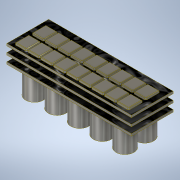
# Autodesk Inventor part: UberDriver_0
Saved by Autodesk Inventor 2020 (Build 240168000, 168)
## iProperties
Created: 2019-02-21
Part Number: UberDriver_0
Material: Silver
Document SubType Name: Modeling
Designer: atmat
Density: 10.49 g/cm^3
Appearance: Silver
Mass: 97.9587 g
Surface Area: 98.3282 cm^2
Volume: 9.3383 cm^3
Author: atmat
Autodesk Inventor part; units mm, degrees
ref_plane "YZ Plane" through (0, 0, 0) normal (1, 0, 0) x (0, 1, 0)
ref_plane "XZ Plane" through (0, 0, 0) normal (0, 1, 0) x (-1, 0, 0)
ref_plane "XY Plane" through (0, 0, 0) normal (0, 0, 1) x (1, 0, 0)
sketch "Szkic1" plane through (0, 0, 0) normal (0, 1, 0) x (-1, 0, 0)
  line L0 (27.94, 9.365) -> (-27.94, 9.365)
  line L1 (-27.94, 9.365) -> (-27.94, -9.365)
  line L2 (-27.94, -9.365) -> (27.94, -9.365)
  line L3 (27.94, -9.365) -> (27.94, 9.365)
  point P0 (0, 0)
  dimension "d0" = 18.73
  dimension "d1" = 9.365
  dimension "d2" = 55.88
  dimension "d3" = 27.94
  constraints: 8 end point, 2 parallel, 1 horizontal, 1 perpendicular
  measures "d0" distance of L2.end L0.start
  measures "d1" distance from line of L0 point (0, 0)
  measures "d2" distance of L0.start L0.end
  measures "d3" distance from line of point (0, 0) L3
extrude "Wyciągnięcie proste1" add sketch "Szkic1" along normal blind 1
sketch "Szkic2" plane through (0, 1, 0) normal (0, 1, 0) x (1, 0, 0)
  line L0 (-25.4, -8.095) -> (-20.32, -8.095)
  line L1 (-20.32, -8.095) -> (-20.32, -2.065)
  line L2 (-20.32, -2.065) -> (-25.4, -2.065)
  line L3 (-25.4, -2.065) -> (-25.4, -8.095)
  line L4 (-27.94, 9.365) -> (-27.94, -9.365) projected
  line L5 (-27.94, -9.365) -> (27.94, -9.365) projected
  line L6 (-19.68, -8.095) -> (-14.6, -8.095)
  line L7 (-14.6, -8.095) -> (-14.6, -2.065)
  line L8 (-14.6, -2.065) -> (-19.68, -2.065)
  line L9 (-19.68, -2.065) -> (-19.68, -8.095)
  line L10 (-13.96, -8.095) -> (-8.88, -8.095)
  line L11 (-8.88, -8.095) -> (-8.88, -2.065)
  line L12 (-8.88, -2.065) -> (-13.96, -2.065)
  line L13 (-13.96, -2.065) -> (-13.96, -8.095)
  line L14 (-8.24, -8.095) -> (-3.16, -8.095)
  line L15 (-3.16, -8.095) -> (-3.16, -2.065)
  line L16 (-3.16, -2.065) -> (-8.24, -2.065)
  line L17 (-8.24, -2.065) -> (-8.24, -8.095)
  line L18 (-2.52, -8.095) -> (2.56, -8.095)
  line L19 (2.56, -8.095) -> (2.56, -2.065)
  line L20 (2.56, -2.065) -> (-2.52, -2.065)
  line L21 (-2.52, -2.065) -> (-2.52, -8.095)
  line L22 (3.2, -8.095) -> (8.28, -8.095)
  line L23 (8.28, -8.095) -> (8.28, -2.065)
  line L24 (8.28, -2.065) -> (3.2, -2.065)
  line L25 (3.2, -2.065) -> (3.2, -8.095)
  line L26 (8.92, -8.095) -> (14, -8.095)
  line L27 (14, -8.095) -> (14, -2.065)
  line L28 (14, -2.065) -> (8.92, -2.065)
  line L29 (8.92, -2.065) -> (8.92, -8.095)
  line L30 (14.64, -8.095) -> (19.72, -8.095)
  line L31 (19.72, -8.095) -> (19.72, -2.065)
  line L32 (19.72, -2.065) -> (14.64, -2.065)
  line L33 (14.64, -2.065) -> (14.64, -8.095)
  line L34 (20.36, -8.095) -> (25.44, -8.095)
  line L35 (25.44, -8.095) -> (25.44, -2.065)
  line L36 (25.44, -2.065) -> (20.36, -2.065)
  line L37 (20.36, -2.065) -> (20.36, -8.095)
  line L38 (-25.4, -0.475) -> (-20.32, -0.475)
  line L39 (-20.32, -0.475) -> (-20.32, 5.555)
  line L40 (-20.32, 5.555) -> (-25.4, 5.555)
  line L41 (-25.4, 5.555) -> (-25.4, -0.475)
  line L42 (-19.68, -0.475) -> (-14.6, -0.475)
  line L43 (-14.6, -0.475) -> (-14.6, 5.555)
  line L44 (-14.6, 5.555) -> (-19.68, 5.555)
  line L45 (-19.68, 5.555) -> (-19.68, -0.475)
  line L46 (-13.96, -0.475) -> (-8.88, -0.475)
  line L47 (-8.88, -0.475) -> (-8.88, 5.555)
  line L48 (-8.88, 5.555) -> (-13.96, 5.555)
  line L49 (-13.96, 5.555) -> (-13.96, -0.475)
  line L50 (19.72, 5.555) -> (14.64, 5.555)
  line L51 (19.72, -0.475) -> (19.72, 5.555)
  line L52 (14.64, -0.475) -> (19.72, -0.475)
  line L53 (14.64, 5.555) -> (14.64, -0.475)
  line L54 (25.44, 5.555) -> (20.36, 5.555)
  line L55 (25.44, -0.475) -> (25.44, 5.555)
  line L56 (20.36, -0.475) -> (25.44, -0.475)
  line L57 (20.36, 5.555) -> (20.36, -0.475)
  line L58 (-3.16, 5.555) -> (-8.24, 5.555)
  line L59 (-3.16, -0.475) -> (-3.16, 5.555)
  line L60 (-8.24, -0.475) -> (-3.16, -0.475)
  line L61 (-8.24, 5.555) -> (-8.24, -0.475)
  line L62 (2.56, 5.555) -> (-2.52, 5.555)
  line L63 (2.56, -0.475) -> (2.56, 5.555)
  line L64 (-2.52, -0.475) -> (2.56, -0.475)
  line L65 (-2.52, 5.555) -> (-2.52, -0.475)
  line L66 (8.28, 5.555) -> (3.2, 5.555)
  line L67 (8.28, -0.475) -> (8.28, 5.555)
  line L68 (3.2, -0.475) -> (8.28, -0.475)
  line L69 (3.2, 5.555) -> (3.2, -0.475)
  line L70 (14, 5.555) -> (8.92, 5.555)
  line L71 (14, -0.475) -> (14, 5.555)
  line L72 (8.92, -0.475) -> (14, -0.475)
  line L73 (8.92, 5.555) -> (8.92, -0.475)
  point P0 (0, 0)
  dimension "d6" = 6.03
  dimension "d7" = 5.08
  dimension "d8" = 2.54
  dimension "d9" = 1.27
  dimension "d10" = 5.08
  dimension "d11" = 6.03
  dimension "d12" = 1.27
  dimension "d13" = 0.64
  dimension "d14" = 5.08
  dimension "d15" = 6.03
  dimension "d16" = 1.27
  dimension "d17" = 0.64
  dimension "d18" = 5.08
  dimension "d19" = 6.03
  dimension "d20" = 1.27
  dimension "d21" = 0.64
  dimension "d22" = 5.08
  dimension "d23" = 6.03
  dimension "d24" = 1.27
  dimension "d25" = 0.64
  dimension "d26" = 5.08
  dimension "d27" = 6.03
  dimension "d28" = 5.08
  dimension "d29" = 6.03
  dimension "d30" = 5.08
  dimension "d31" = 6.03
  dimension "d32" = 5.08
  dimension "d33" = 6.03
  dimension "d34" = 0.64
  dimension "d35" = 0.64
  dimension "d36" = 0.64
  dimension "d37" = 0.64
  dimension "d38" = 1.27
  dimension "d39" = 1.27
  dimension "d40" = 1.27
  dimension "d41" = 1.27
  dimension "d42" = 6.03
  dimension "d43" = 5.08
  dimension "d44" = 6.03
  dimension "d45" = 5.08
  dimension "d46" = 6.03
  dimension "d47" = 5.08
  dimension "d48" = 1.59
  dimension "d49" = 0
  dimension "d50" = 0
  dimension "d51" = 0
  dimension "d52" = 0
  dimension "d53" = 0
  dimension "d54" = 5.08
  dimension "d55" = 6.03
  dimension "d56" = 5.08
  dimension "d57" = 6.03
  dimension "d58" = 0.64
  dimension "d59" = 0
  dimension "d60" = 0
  dimension "d61" = 0
  dimension "d62" = 5.08
  dimension "d63" = 6.03
  dimension "d64" = 5.08
  dimension "d65" = 6.03
  dimension "d66" = 0.64
  dimension "d67" = 0
  dimension "d68" = 0
  dimension "d69" = 0
  constraints: 144 end point, 36 parallel, 18 horizontal, 18 perpendicular
  measures "d6" distance of L2.end L0.start
  measures "d7" distance of L1.end L2.end
  measures "d8" distance between parallel lines of L4 L3
  measures "d9" distance between parallel lines of L5 L0
  measures "d10" distance of L7.end L8.end
  measures "d11" distance of L8.end L6.start
  measures "d12" distance between parallel lines of L5 L6
  measures "d13" distance between parallel lines of L9 L1
  measures "d14" distance of L12.start L12.end
  measures "d15" distance of L12.end L10.start
  measures "d16" distance between parallel lines of L5 L10
  measures "d17" distance between parallel lines of L13 L7
  measures "d18" distance of L16.start L16.end
  measures "d19" distance of L16.end L14.start
  measures "d20" distance between parallel lines of L14 L5
  measures "d21" distance between parallel lines of L11 L17
  measures "d22" distance of L20.start L20.end
  measures "d23" distance of L20.end L18.start
  measures "d24" distance between parallel lines of L5 L18
  measures "d25" distance between parallel lines of L15 L21
  measures "d26" distance of L24.start L24.end
  measures "d27" distance of L24.end L22.start
  measures "d28" distance of L28.start L28.end
  measures "d29" distance of L28.end L26.start
  measures "d30" distance of L32.start L32.end
  measures "d31" distance of L32.end L30.start
  measures "d32" distance of L36.start L36.end
  measures "d33" distance of L36.end L34.start
  measures "d34" distance between parallel lines of L25 L19
  measures "d35" distance between parallel lines of L29 L23
  measures "d36" distance between parallel lines of L33 L27
  measures "d37" distance between parallel lines of L37 L31
  measures "d38" distance between parallel lines of L5 L22
  measures "d39" distance between parallel lines of L5 L26
  measures "d40" distance between parallel lines of L5 L30
  measures "d41" distance between parallel lines of L5 L34
  measures "d42" distance of L40.end L38.start
  measures "d43" distance of L39.end L40.end
  measures "d44" distance of L44.end L42.start
  measures "d45" distance of L43.end L44.end
  measures "d46" distance of L48.end L46.start
  measures "d47" distance of L47.end L48.end
  measures "d48" distance between parallel lines of L38 L2
  measures "d49" distance between parallel lines of L3 L41
  measures "d50" distance between parallel lines of L9 L45
  measures "d51" distance between parallel lines of L13 L49
  measures "d52" distance between parallel lines of L38 L42
  measures "d53" distance between parallel lines of L42 L46
  measures "d54" distance of L50.start L53.start
  measures "d55" distance of L53.start L53.end
  measures "d56" distance of L54.start L57.start
  measures "d57" distance of L57.start L57.end
  measures "d58" distance between parallel lines of L57 L51
  measures "d59" distance between parallel lines of L52 L46
  measures "d60" distance between parallel lines of L52 L56
  measures "d61" distance between parallel lines of L37 L57
  measures "d62" distance of L58.start L61.start
  measures "d63" distance of L61.start L61.end
  measures "d64" distance of L62.start L65.start
  measures "d65" distance of L65.start L65.end
  measures "d66" distance between parallel lines of L65 L59
  measures "d67" distance between parallel lines of L58 L62
  measures "d68" distance between parallel lines of L19 L63
  measures "d69" distance between parallel lines of L48 L58
extrude "Wyciągnięcie proste2" add sketch "Szkic2" along normal blind 1
chamfer "Faza1" distance 0.2 angle 45 4 edges at (22.9, 2, 8.095) (25.44, 2, 5.08) (20.36, 2, 5.08) (22.9, 2, 2.065)
chamfer "Faza2" distance 0.2 angle 45 68 edges at (17.18, 2, 8.095) (19.72, 2, 5.08) (14.64, 2, 5.08) (17.18, 2, 2.065) (14, 2, 5.08) (11.46, 2, 8.095) (8.92, 2, 5.08) (11.46, 2, 2.065) (8.28, 2, 5.08) (5.74, 2, 8.095) (3.2, 2, 5.08) (5.74, 2, 2.065) (0.02, 2, 8.095) (-5.7, 2, 8.095) (-11.42, 2, 8.095) (-17.14, 2, 8.095) (-22.86, 2, 8.095) (-25.4, 2, 5.08) (-22.86, 2, 2.065) (-17.14, 2, 2.065) (-19.68, 2, 5.08) (-14.6, 2, 5.08) (-13.96, 2, 5.08) (-8.88, 2, 5.08) (-11.42, 2, 2.065) (-5.7, 2, 2.065) (-3.16, 2, 5.08) (-8.24, 2, 5.08) (-20.32, 2, 5.08) (-20.32, 2, -2.54) (-22.86, 2, 0.475) (-25.4, 2, -2.54) (-22.86, 2, -5.555) (-17.14, 2, -5.555) (-19.68, 2, -2.54) (-17.14, 2, 0.475) (-14.6, 2, -2.54) (-11.42, 2, 0.475) (-13.96, 2, -2.54) (-11.42, 2, -5.555) (-8.88, 2, -2.54) (-5.7, 2, 0.475) (-8.24, 2, -2.54) (-5.7, 2, -5.555) (-3.16, 2, -2.54) (0.02, 2, 2.065) (-2.52, 2, 5.08) (0.02, 2, 0.475) (-2.52, 2, -2.54) (0.02, 2, -5.555) (2.56, 2, -2.54) (5.74, 2, 0.475) (3.2, 2, -2.54) (5.74, 2, -5.555) (8.28, 2, -2.54) (11.46, 2, 0.475) (8.92, 2, -2.54) (11.46, 2, -5.555) (14, 2, -2.54) (17.18, 2, 0.475) (17.18, 2, -5.555) (14.64, 2, -2.54) (19.72, 2, -2.54) (22.9, 2, 0.475) (20.36, 2, -2.54) (22.9, 2, -5.555) (25.44, 2, -2.54) (2.56, 2, 5.08)
chamfer "Faza3" distance 0.5 angle 45 18 edges at (25.44, 1.4, 8.095) (19.72, 1.4, 8.095) (14, 1.4, 8.095) (8.28, 1.4, 8.095) (2.56, 1.4, 8.095) (2.56, 1.4, 0.475) (8.28, 1.4, 0.475) (14, 1.4, 0.475) (19.72, 1.4, 0.475) (25.44, 1.4, 0.475) (-3.16, 1.4, 0.475) (-3.16, 1.4, 8.095) (-8.88, 1.4, 8.095) (-14.6, 1.4, 8.095) (-8.88, 1.4, 0.475) (-14.6, 1.4, 0.475) (-20.32, 1.4, 0.475) (-20.32, 1.4, 8.095)
sketch "Szkic3" plane through (0, 0, 0) normal (0, -1, 0) x (1, 0, 0)
  line L0 (-25.08, -2.085) -> (-21.9, -2.085)
  line L1 (-21.9, -2.085) -> (-21.9, -8.435)
  line L2 (-21.9, -8.435) -> (-25.08, -8.435)
  line L3 (-25.08, -8.435) -> (-25.08, -2.085)
  line L4 (-25.4, 0.475) -> (-25.4, -5.555) projected
  line L5 (27.94, -9.365) -> (-27.94, -9.365) projected
  line L6 (-19.36, -2.085) -> (-16.18, -2.085)
  line L7 (-16.18, -2.085) -> (-16.18, -8.435)
  line L8 (-16.18, -8.435) -> (-19.36, -8.435)
  line L9 (-19.36, -8.435) -> (-19.36, -2.085)
  line L10 (-19.68, 0.475) -> (-19.68, -5.555) projected
  line L11 (-13.64, -2.085) -> (-10.46, -2.085)
  line L12 (-10.46, -2.085) -> (-10.46, -8.435)
  line L13 (-10.46, -8.435) -> (-13.64, -8.435)
  line L14 (-13.64, -8.435) -> (-13.64, -2.085)
  line L15 (-7.92, -2.085) -> (-4.74, -2.085)
  line L16 (-4.74, -2.085) -> (-4.74, -8.435)
  line L17 (-4.74, -8.435) -> (-7.92, -8.435)
  line L18 (-7.92, -8.435) -> (-7.92, -2.085)
  line L19 (-2.2, -2.085) -> (0.98, -2.085)
  line L20 (0.98, -2.085) -> (0.98, -8.435)
  line L21 (0.98, -8.435) -> (-2.2, -8.435)
  line L22 (-2.2, -8.435) -> (-2.2, -2.085)
  line L23 (3.52, -2.085) -> (6.7, -2.085)
  line L24 (6.7, -2.085) -> (6.7, -8.435)
  line L25 (6.7, -8.435) -> (3.52, -8.435)
  line L26 (3.52, -8.435) -> (3.52, -2.085)
  line L27 (9.24, -2.085) -> (12.42, -2.085)
  line L28 (12.42, -2.085) -> (12.42, -8.435)
  line L29 (12.42, -8.435) -> (9.24, -8.435)
  line L30 (9.24, -8.435) -> (9.24, -2.085)
  line L31 (14.96, -8.435) -> (14.96, -2.085)
  line L32 (14.96, -2.085) -> (18.14, -2.085)
  line L33 (18.14, -2.085) -> (18.14, -8.435)
  line L34 (18.14, -8.435) -> (14.96, -8.435)
  line L35 (20.68, -8.435) -> (20.68, -2.085)
  line L36 (20.68, -2.085) -> (23.86, -2.085)
  line L37 (23.86, -2.085) -> (23.86, -8.435)
  line L38 (23.86, -8.435) -> (20.68, -8.435)
  point P0 (0, 0)
  dimension "d89" = 6.35
  dimension "d90" = 3.18
  dimension "d91" = 0.32
  dimension "d92" = 0.93
  dimension "d93" = 6.35
  dimension "d94" = 3.18
  dimension "d95" = 0.32
  dimension "d96" = 0
  dimension "d97" = 6.35
  dimension "d98" = 3.18
  dimension "d99" = 2.54
  dimension "d100" = 0
  dimension "d101" = 6.35
  dimension "d102" = 3.18
  dimension "d103" = 6.35
  dimension "d104" = 3.18
  dimension "d105" = 6.35
  dimension "d106" = 3.18
  dimension "d107" = 6.35
  dimension "d108" = 3.18
  dimension "d109" = 0
  dimension "d110" = 0
  dimension "d111" = 2.54
  dimension "d112" = 2.54
  dimension "d113" = 2.54
  dimension "d114" = 2.54
  dimension "d115" = 6.35
  dimension "d116" = 3.18
  dimension "d117" = 6.35
  dimension "d118" = 3.18
  dimension "d119" = 2.54
  dimension "d120" = 2.54
  constraints: 72 end point, 18 parallel, 9 horizontal, 9 perpendicular, 4 collinear
  measures "d89" distance of L0.end L1.end
  measures "d90" distance of L0.start L0.end
  measures "d91" distance between parallel lines of L3 L4
  measures "d92" distance between parallel lines of L2 L5
  measures "d93" distance of L6.end L7.end
  measures "d94" distance of L9.end L6.end
  measures "d95" distance between parallel lines of L10 L9
  measures "d96" distance between parallel lines of L2 L8
  measures "d97" distance of L11.end L12.end
  measures "d98" distance of L14.end L11.end
  measures "d99" distance between parallel lines of L7 L14
  measures "d100" distance between parallel lines of L6 L11
  measures "d101" distance of L15.end L16.end
  measures "d102" distance of L18.end L15.end
  measures "d103" distance of L19.end L20.end
  measures "d104" distance of L22.end L19.end
  measures "d105" distance of L23.end L24.end
  measures "d106" distance of L26.end L23.end
  measures "d107" distance of L27.end L28.end
  measures "d108" distance of L30.end L27.end
  measures "d109" distance between parallel lines of L13 L17
  measures "d110" distance between parallel lines of L17 L21
  measures "d111" distance between parallel lines of L12 L18
  measures "d112" distance between parallel lines of L16 L22
  measures "d113" distance between parallel lines of L26 L20
  measures "d114" distance between parallel lines of L30 L24
  measures "d115" distance of L32.end L34.start
  measures "d116" distance of L31.end L32.end
  measures "d117" distance of L37.start L38.start
  measures "d118" distance of L35.end L37.start
  measures "d119" distance between parallel lines of L35 L33
  measures "d120" distance between parallel lines of L28 L31
extrude "Wyciągnięcie proste3" add sketch "Szkic3" along normal blind 0.35
chamfer "Faza4" distance 0.35 angle 45 18 edges at (22.27, -0.35, -2.085) (16.55, -0.35, -2.085) (10.83, -0.35, -2.085) (5.11, -0.35, -2.085) (-0.61, -0.35, -2.085) (-6.33, -0.35, -2.085) (-12.05, -0.35, -2.085) (-17.77, -0.35, -2.085) (-23.49, -0.35, -2.085) (-23.49, -0.35, -8.435) (-17.77, -0.35, -8.435) (-12.05, -0.35, -8.435) (-6.33, -0.35, -8.435) (-0.61, -0.35, -8.435) (5.11, -0.35, -8.435) (10.83, -0.35, -8.435) (16.55, -0.35, -8.435) (22.27, -0.35, -8.435)
sketch "Szkic4" plane through (0, 0, 0) normal (0, -1, 0) x (1, 0, 0)
  line L0 (-16.32, -0.535) -> (-13.32, -0.535)
  line L1 (-13.32, -0.535) -> (-13.32, -1.935)
  line L2 (-13.32, -1.935) -> (-16.32, -1.935)
  line L3 (-16.32, -1.935) -> (-16.32, -0.535)
  line L4 (-25.08, -2.085) -> (-21.9, -2.085) projected
  line L5 (-10.46, -8.085) -> (-10.46, -2.435) projected
  line L6 (0.84, -0.535) -> (3.84, -0.535)
  line L7 (3.84, -0.535) -> (3.84, -1.935)
  line L8 (3.84, -1.935) -> (0.84, -1.935)
  line L9 (0.84, -1.935) -> (0.84, -0.535)
  line L10 (6.7, -8.085) -> (6.7, -2.435) projected
  line L11 (-2.2, -2.085) -> (0.98, -2.085) projected
  line L12 (18, -0.535) -> (21, -0.535)
  line L13 (21, -0.535) -> (21, -1.935)
  line L14 (21, -1.935) -> (18, -1.935)
  line L15 (18, -1.935) -> (18, -0.535)
  line L16 (23.86, -8.085) -> (23.86, -2.435) projected
  line L17 (14.96, -2.085) -> (18.14, -2.085) projected
  point P0 (0, 0)
  dimension "d126" = 1.4
  dimension "d127" = 3
  dimension "d128" = 0.15
  dimension "d129" = 2.86
  dimension "d130" = 1.4
  dimension "d131" = 3
  dimension "d132" = 2.86
  dimension "d133" = 0.15
  dimension "d134" = 1.4
  dimension "d135" = 3
  dimension "d136" = 2.86
  dimension "d137" = 0.15
  constraints: 24 end point, 6 parallel, 3 horizontal, 3 perpendicular
  measures "d126" distance of L2.end L0.start
  measures "d127" distance of L0.start L0.end
  measures "d128" distance between parallel lines of L4 L2
  measures "d129" distance between parallel lines of L1 L5
  measures "d130" distance of L8.end L6.start
  measures "d131" distance of L6.start L6.end
  measures "d132" distance between parallel lines of L10 L7
  measures "d133" distance between parallel lines of L11 L8
  measures "d134" distance of L14.end L12.start
  measures "d135" distance of L12.start L12.end
  measures "d136" distance between parallel lines of L13 L16
  measures "d137" distance between parallel lines of L17 L14
extrude "Wyciągnięcie proste4" add sketch "Szkic4" along normal blind 1.1
chamfer "Faza5" distance 0.6 angle 25 1 edges at (-14.82, -1.1, -0.535) measured on face at (-15.32, -0.3667, -0.535)
chamfer "Faza6" distance 0.6 angle 25 1 edges at (2.34, -1.1, -0.535) measured on face at (1.84, -0.3667, -0.535)
chamfer "Faza7" distance 0.6 angle 25 1 edges at (19.5, -1.1, -0.535) measured on face at (19, -0.3667, -0.535)
chamfer "Faza8" distance 0.6 angle 25 1 edges at (19.5, -1.1, -1.935) measured on face at (20, -0.3667, -1.935)
chamfer "Faza9" distance 0.6 angle 25 1 edges at (2.34, -1.1, -1.935) measured on face at (2.84, -0.3667, -1.935)
chamfer "Faza10" distance 0.6 angle 25 1 edges at (-14.82, -1.1, -1.935) measured on face at (-14.32, -0.3667, -1.935)
chamfer "Faza11" distance 0.6 angle 25 1 edges at (-13.32, -1.1, -1.235) measured on face at (-13.32, -0.7, -1.0949)
chamfer "Faza12" distance 0.6 angle 25 1 edges at (3.84, -1.1, -1.235) measured on face at (3.84, -0.7, -1.0949)
chamfer "Faza13" distance 0.6 angle 25 1 edges at (21, -1.1, -1.235) measured on face at (21, -0.7, -1.0949)
chamfer "Faza14" distance 0.6 angle 25 1 edges at (18, -1.1, -1.235) measured on face at (18, -0.7, -1.3751)
chamfer "Faza15" distance 0.6 angle 25 1 edges at (0.84, -1.1, -1.235) measured on face at (0.84, -0.7, -1.3751)
chamfer "Faza16" distance 0.6 angle 25 1 edges at (-16.32, -1.1, -1.235) measured on face at (-16.32, -0.7, -1.3751)
ref_plane "Płaszczyzna konstrukcyjna1" through (0, -3.55, 0) normal (0, -1, 0) x (1, 0, 0)
sketch "Szkic5" plane through (0, -3.55, 0) normal (0, -1, 0) x (1, 0, 0)
  line L0 (-22.54, 4.285) -> (-15.54, 4.285)
  line L1 (-15.54, 4.285) -> (-15.54, -2.715)
  line L2 (-15.54, -2.715) -> (-22.54, -2.715)
  line L3 (-22.54, -2.715) -> (-22.54, 4.285)
  line L4 (-27.94, -9.365) -> (-27.94, 9.365) projected
  line L5 (-27.94, 9.365) -> (27.94, 9.365) projected
  line L6 (-3.5, 4.285) -> (3.5, 4.285)
  line L7 (3.5, 4.285) -> (3.5, -2.715)
  line L8 (3.5, -2.715) -> (-3.5, -2.715)
  line L9 (-3.5, -2.715) -> (-3.5, 4.285)
  line L10 (15.54, 4.285) -> (22.54, 4.285)
  line L11 (22.54, 4.285) -> (22.54, -2.715)
  line L12 (22.54, -2.715) -> (15.54, -2.715)
  line L13 (15.54, -2.715) -> (15.54, 4.285)
  line L14 (27.94, 9.365) -> (27.94, -9.365) projected
  point P0 (0, 0)
  dimension "d177" = 7
  dimension "d178" = 7
  dimension "d179" = 5.4
  dimension "d180" = 5.08
  dimension "d181" = 7
  dimension "d182" = 7
  dimension "d183" = 7
  dimension "d184" = 7
  dimension "d185" = 5.4
  dimension "d186" = 0
  dimension "d187" = 0
  dimension "d188" = 3.5
  constraints: 24 end point, 6 parallel, 3 horizontal, 3 perpendicular
  measures "d177" distance of L0.start L0.end
  measures "d178" distance of L0.end L1.end
  measures "d179" distance between parallel lines of L4 L3
  measures "d180" distance between parallel lines of L5 L0
  measures "d181" distance of L6.start L6.end
  measures "d182" distance of L6.end L7.end
  measures "d183" distance of L10.start L10.end
  measures "d184" distance of L10.end L11.end
  measures "d185" distance between parallel lines of L14 L11
  measures "d186" distance between parallel lines of L6 L10
  measures "d187" distance between parallel lines of L6 L0
  measures "d188" distance from line of L9 point (0, 0)
extrude "Wyciągnięcie proste5" add sketch "Szkic5" along normal blind 1
sketch "Szkic6" plane through (0, -3.55, 0) normal (0, 1, 0) x (1, 0, 0)
  line L0 (27.94, 9.365) -> (-27.94, 9.365) projected
  line L1 (-27.94, -9.365) -> (27.94, -9.365) projected
  line L2 (-27.94, 9.365) -> (27.94, 9.365)
  line L3 (27.94, 9.365) -> (27.94, -9.365)
  line L4 (27.94, -9.365) -> (-27.94, -9.365)
  line L5 (-27.94, -9.365) -> (-27.94, 9.365)
  point P0 (0, 0)
  constraints: 8 end point, 2 parallel, 1 horizontal, 1 perpendicular
extrude "Wyciągnięcie proste6" add sketch "Szkic6" along normal blind 1
sketch "Szkic7" plane through (0, -4.55, 0) normal (0, -1, 0) x (1, 0, 0)
  line L0 (-5, 5) -> (5, 5)
  line L1 (5, 5) -> (5, -5)
  line L2 (5, -5) -> (-5, -5)
  line L3 (-5, -5) -> (-5, 5)
  point P0 (0, 0)
  dimension "d193" = 10
  dimension "d194" = 10
  dimension "d195" = 5
  dimension "d196" = 5
  constraints: 8 end point, 2 parallel, 1 horizontal, 1 perpendicular
  measures "d193" distance of L0.end L1.end
  measures "d194" distance of L1.end L2.end
  measures "d195" distance from line of point (0, 0) L1
  measures "d196" distance from line of point (0, 0) L0
extrude "Wyciągnięcie proste7" add sketch "Szkic7" along normal blind 1.6
sketch "Szkic8" plane through (0, -6.15, 0) normal (0, -1, 0) x (1, 0, 0)
  line L0 (27.94, 9.365) -> (27.94, -9.365) projected
  line L1 (27.94, 9.365) -> (-27.94, 9.365) projected
  line L2 (27.94, -9.365) -> (-27.94, -9.365)
  line L3 (-27.94, -9.365) -> (-27.94, 9.365)
  line L4 (-27.94, 9.365) -> (27.94, 9.365)
  line L5 (27.94, 9.365) -> (27.94, -9.365)
  point P0 (0, 0)
  constraints: 8 end point, 2 parallel, 1 horizontal, 1 perpendicular
extrude "Wyciągnięcie proste8" add sketch "Szkic8" along normal blind 1
sketch "Szkic9" plane through (0, -7.15, 0) normal (0, -1, 0) x (1, 0, 0)
  circle A0 centre (20.32, -4.285) radius 4
  circle A1 centre (20.32, 4.605) radius 4
  line L0 (27.94, -9.365) -> (27.94, 9.365) projected
  circle A2 centre (10.16, -4.285) radius 4
  circle A3 centre (10.16, 4.605) radius 4
  circle A4 centre (0, -4.285) radius 4
  circle A5 centre (-10.16, -4.285) radius 4
  circle A6 centre (-20.32, -4.285) radius 4
  circle A7 centre (0, 4.605) radius 4
  circle A8 centre (-10.16, 4.605) radius 4
  line L1 (-20.32, 7.595) -> (-20.32, 2.065) projected
  circle A9 centre (-20.32, 4.605) radius 4
  line L2 (-27.94, -9.365) -> (27.94, -9.365) projected
  point P0 (0, 0)
  dimension "d201" = 8
  dimension "d202" = 8
  dimension "d203" = 8.89
  dimension "d204" = 7.62
  dimension "d205" = 7.62
  dimension "d206" = 8
  dimension "d207" = 10.16
  dimension "d208" = 0
  dimension "d209" = 8
  dimension "d210" = 8
  dimension "d211" = 8
  dimension "d212" = 8
  dimension "d213" = 10.16
  dimension "d214" = 10.16
  dimension "d215" = 10.16
  dimension "d216" = 8
  dimension "d217" = 8
  dimension "d218" = 8
  dimension "d219" = 5.08
  dimension "d220" = 0
  dimension "d221" = 0
  dimension "d222" = 0
  dimension "d223" = 0
  constraints: 10 centre point, 1 point on line
  measures "d201" diameter of A0
  measures "d202" diameter of A1
  measures "d203" distance of A1.centre A0.centre
  measures "d204" distance from line of L0 A0.centre
  measures "d205" distance from line of L0 A1.centre
  measures "d206" diameter of A2
  measures "d207" distance of A2.centre A0.centre
  measures "d208" vertical distance of A0.centre A2.centre
  measures "d209" diameter of A3
  measures "d210" diameter of A4
  measures "d211" diameter of A5
  measures "d212" diameter of A6
  measures "d213" distance of A2.centre A4.centre
  measures "d214" distance of A5.centre A4.centre
  measures "d215" distance of A6.centre A5.centre
  measures "d216" diameter of A7
  measures "d217" diameter of A8
  measures "d218" diameter of A9
  measures "d219" distance from line of L2 A0.centre
  measures "d220" vertical distance of A1.centre A3.centre
  measures "d221" vertical distance of A3.centre A7.centre
  measures "d222" vertical distance of A1.centre A8.centre
  measures "d223" vertical distance of A1.centre A9.centre
extrude "Wyciągnięcie proste9" add sketch "Szkic9" along normal blind 10.5
